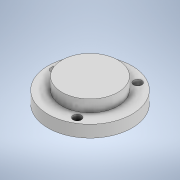
# Autodesk Inventor part: 7.1 Part 6
Saved by Autodesk Inventor 2020 (Build 240168000, 168)
## iProperties
Created: 2020-03-13
Part Number: 7.1 Part 6
Material: Generic
Document SubType Name: Modeling
Designer: cks4a449
Density: 1 g/cm^3
Appearance: Default
Author: cks4a449
Autodesk Inventor part; units mm, degrees
ref_plane "YZ Plane" through (0, 0, 0) normal (1, 0, 0) x (0, 1, 0)
ref_plane "XZ Plane" through (0, 0, 0) normal (0, 1, 0) x (-1, 0, 0)
ref_plane "XY Plane" through (0, 0, 0) normal (0, 0, 1) x (1, 0, 0)
sketch "Sketch1" plane through (0, 0, 0) normal (0, 1, 0) x (-1, 0, 0)
  circle A0 centre (0, 0) radius 22.225
  circle A1 centre (0, 0) radius 14.7955
  line L0 (22.225, 0) -> (14.7955, 0)
  circle A2 centre (18.5103, 0) radius 2.1844
  circle A3 centre (-9.2551, 16.0303) radius 2.1844
  circle A4 centre (-9.2551, -16.0303) radius 2.1844
  dimension "d0" = 44.45
  dimension "d1" = 29.591
  dimension "d2" = 4.3688
  dimension "d5" = 360
  constraints: 3 centre point, 2 coincident, 2 end point, 2 horizontal alignment, 1 horizontal, 1 midpoint, 11 other
  measures "d2" diameter of A2
extrude "Extrusion1" add sketch "Sketch1" along normal blind 6.35
extrude "Extrusion2" add sketch "Sketch1" along normal blind 12.7 contours A1
body "Solid1"
